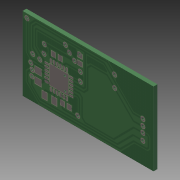
# Autodesk Inventor part: GPS_module_PCB
Saved by Autodesk Inventor 2013 (Build 170138000, 138)
## iProperties
Created: 2015-07-02
Part Number: GPS_module_PCB
Material: Ogólny
Document SubType Name: Modeling
Designer: terg
Density: 1 g/cm^3
Author: terg
Autodesk Inventor part; units mm, degrees
ref_plane "YZ Plane" through (0, 0, 0) normal (1, 0, 0) x (0, 1, 0)
ref_plane "XZ Plane" through (0, 0, 0) normal (0, 1, 0) x (-1, 0, 0)
ref_plane "XY Plane" through (0, 0, 0) normal (0, 0, 1) x (1, 0, 0)
sketch "Szkic1" plane through (0, 0, 0) normal (0, 1, 0) x (-1, 0, 0)
  line L0 (0, 0) -> (26.75, 0)
  line L1 (26.75, 0) -> (26.75, 15)
  line L2 (26.75, 15) -> (0, 15)
  line L3 (0, 15) -> (0, 0)
  dimension "d0" = 26.75
  dimension "d1" = 15
  constraints: 8 end point, 2 parallel, 1 horizontal, 1 perpendicular
  measures "d0" distance of L2.end L1.end
  measures "d1" distance of L1.end L0.end
extrude "Wyciągnięcie proste1" add sketch "Szkic1" along normal blind 0.8
sketch "Szkic2" plane through (0, 0.8, 0) normal (0, 1, 0) x (1, 0, 0)
  line L0 (0, 0) -> (-26.75, 0) projected
  line L1 (-26.75, 0) -> (-26.75, -15) projected
  line L2 (-26.75, -15) -> (0, -15) projected
  line L3 (0, -15) -> (0, 0) projected
  line L4 (-26.6405, 0) -> (-0.1095, 0) construction
  line L5 (-0.1095, 0) -> (-0.1095, -15) construction
  line L6 (-0.1095, -15) -> (-26.6405, -15) construction
  line L7 (-26.6405, -15) -> (-26.6405, 0) construction
  dimension "d9" = 0
  dimension "d10" = 0.1095
  dimension "d11" = 0
  dimension "d12" = 0.1095
  constraints: 2 other
  measures "d9" distance between parallel lines of L0 L4
  measures "d10" distance between parallel lines of L3 L5
  measures "d11" distance between parallel lines of L2 L6
  measures "d12" distance between parallel lines of L1 L7
decal "Pokrycie bitmapą1"
sketch "Szkic3" plane through (0, 0, 0) normal (0, -1, 0) x (1, 0, 0)
  line L0 (0, 0) -> (-26.75, 0) projected
  line L1 (0, 15) -> (0, 0) projected
  line L2 (-26.75, 15) -> (0, 15) projected
  line L3 (-26.75, 0) -> (-26.75, 15) projected
  line L4 (-0.0767, 0) -> (-26.6733, 0) construction
  line L5 (-26.6733, 0) -> (-26.6733, 15) construction
  line L6 (-26.6733, 15) -> (-0.0767, 15) construction
  line L7 (-0.0767, 15) -> (-0.0767, 0) construction
  dimension "d19" = 0
  dimension "d21" = 0.0767
  dimension "d22" = 0
  dimension "d23" = 0.0767
  constraints: 2 other
  measures "d19" distance between parallel lines of L0 L4
  measures "d21" distance between parallel lines of L1 L7
  measures "d22" distance between parallel lines of L2 L6
  measures "d23" distance between parallel lines of L3 L5
decal "Pokrycie bitmapą2"
sketch "Szkic4" plane through (0, 0, 0) normal (0, -1, 0) x (1, 0, 0)
  point P0 (-25.8651, 14.1572)
  point P1 (-18.0182, 13.3937)
  point P2 (-17.1982, 12.4182)
  point P3 (-16.1519, 11.4709)
  point P4 (-15.1056, 13.1393)
  point P5 (-22.3163, 11.3578)
  point P6 (-22.3833, 9.6174)
  point P7 (-14.9594, 10.1441)
  point P8 (-14.9594, 8.3784)
  point P9 (-24.6782, 8.4428)
  point P10 (-23.2134, 8.1772)
  point P11 (-25.0646, 6.6882)
  point P12 (-24.807, 5.5694)
  point P13 (-24.8875, 4.3782)
  point P14 (-15.4719, 2.0939)
  point P15 (-7.9556, 13.1393)
  point P16 (-7.9556, 10.7325)
  point P17 (-2.1744, 8.1772)
  point P18 (-2.1744, 6.9068)
  point P19 (-2.1744, 5.735)
  point P20 (-2.219, 4.3244)
  point P21 (-18.0182, 5.1433)
  point P22 (-18.1375, 7.8541)
hole "Otwór1" at (-25.8651, 0, 14.1572) at (-18.0182, 0, 13.3937) at (-17.1982, 0, 12.4182) at (-16.1519, 0, 11.4709) at (-15.1056, 0, 13.1393) at (-22.3163, 0, 11.3578) at (-22.3833, 0, 9.6174) at (-14.9594, 0, 10.1441) at (-14.9594, 0, 8.3784) at (-24.6782, 0, 8.4428) at (-23.2134, 0, 8.1772) at (-25.0646, 0, 6.6882) at (-24.807, 0, 5.5694) at (-24.8875, 0, 4.3782) at (-15.4719, 0, 2.0939) at (-7.9556, 0, 13.1393) at (-7.9556, 0, 10.7325) at (-2.1744, 0, 8.1772) at (-2.1744, 0, 6.9068) at (-2.1744, 0, 5.735) at (-2.219, 0, 4.3244) at (-18.0182, 0, 5.1433) at (-18.1375, 0, 7.8541) direction (0, 1, 0) diameter 0.4 depth 8
equation "\"d10\" = d12"
equation "\"d21\" = d23"
